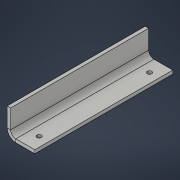
# Autodesk Inventor part: 200512
Saved by Autodesk Inventor 2022.2 (Build 262287000, 287)
## iProperties
Created: 2022-08-22
Part Number: 200512
Material: Aluminum 5052 H32
Document SubType Name: Sheet Metal
Designer: robotics
Mass: 48.6573 g
Surface Area: 125.251 cm^2
Volume: 18.0212 cm^3
Density: 2.7 g/cm^3
Sheet Metal Rule: .125 5052
Appearance: Aluminum - Flat
Author: robotics
Autodesk Inventor part; units mm, degrees
ref_plane "YZ Plane" through (0, 0, 0) normal (1, 0, 0) x (0, 1, 0)
ref_plane "XZ Plane" through (0, 0, 0) normal (0, 1, 0) x (-1, 0, 0)
ref_plane "XY Plane" through (0, 0, 0) normal (0, 0, 1) x (1, 0, 0)
sketch "Sketch1" plane through (0, 0, 0) normal (0, 1, 0) x (-1, 0, 0)
  line L0 (0, 0) -> (25.4, 0)
  line L1 (25.4, 0) -> (25.4, 127)
  line L2 (25.4, 127) -> (0, 127)
  line L3 (0, 127) -> (0, 0)
  dimension "d0" = 25.4
  dimension "d1" = 127
  measures "d0" distance of L1.end L2.end
  measures "d1" distance of L0.end L1.end
extrude "Plate1" add sketch "Sketch1" along normal blind 3.175
sketch "Sketch2" plane through (-22.225, 0, 127) normal (-1, 0, 0) x (0, -1, 0)
  line L0 (0, -127) -> (0, 0)
  line L1 (0, 0) -> (-25.4, 0)
  line L2 (-25.4, 0) -> (-25.4, -127)
  line L3 (-25.4, -127) -> (0, -127)
  constraints: 6 end point, 1 horizontal, 1 perpendicular, 1 vertical
edge flange "Flange1" height 25.4 angle 90 thickness 3.175 bend radius 4.7625 thickness toward (-1, 0, 0) relief tear relief width 3.175 relief depth 1.5875 edges at (-25.4, 3.175, 63.5) wall of the first edge with corners at (-22.225, 0, 0) (-22.225, 0, 127) (-22.225, 25.4, 127) (-22.225, 25.4, 0)
bend "Bend1"
corner "Corner1"
sketch "Sketch3" plane through (0, 3.175, 0) normal (0, 1, 0) x (1, 0, 0)
  line L0 (-17.4625, 0) -> (0, 0) construction
  line L1 (-8.7313, 0) -> (-8.7312, -127) construction
  line L2 (0, -127) -> (-17.4625, -127) construction
  point P0 (-8.7312, -12.7)
  point P1 (-8.7312, -114.3)
  dimension "d13" = 12.7
  dimension "d14" = 12.7
  constraints: 2 end point, 2 midpoint, 2 point on line
  measures "d13" distance from line of L0 point (-8.731, -12.7)
  measures "d14" distance from line of L2 point (-8.731, -114.3)
hole "Hole1" at (-8.7312, 3.175, 12.7) at (-8.7312, 3.175, 114.3) direction (0, -1, 0) diameter 4.0894 end through all clearance for "Pop Rivet" size "5/32" standard "4859 Fastners"
equation "\"d20\" = Thickness"
equation "\"d2\" = Thickness"
equation "\"d3\" = BendReliefWidth"
equation "\"d4\" = BendReliefDepth"
equation "\"d5\" = MinimumRemnant"
equation "\"d6\" = TransitionRadius"
equation "\"d9\" = BendRadius"
equation "\"d10\" = CornerReliefSize"
equation "\"d11\" = GapSize"
equation "\"d12\" = JacobiRadiusSize"
equation "\"BendRadius\" = 1.5 * Thickness"
equation "\"BendReliefWidth\" = Thickness"
equation "\"BendReliefDepth\" = 0.5 * Thickness"
equation "\"CornerReliefSize\" = 4 * Thickness"
equation "\"MinimumRemnant\" = 2 * Thickness"
equation "\"TransitionRadius\" = BendRadius"
equation "\"JacobiRadiusSize\" = BendRadius"
equation "\"GapSize\" = Thickness"
equation "\"Thickness\" = 3.175"
body "Solid1"
